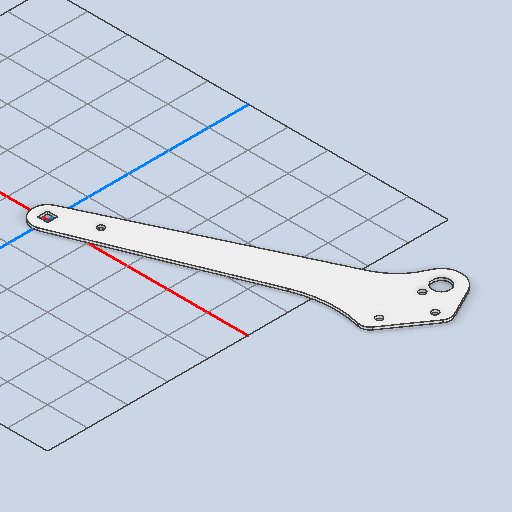
# Autodesk Inventor part: Gusset
Saved by Autodesk Inventor 2026 (Build 300175000, 175)
## iProperties
Created: 2025-04-12
Part Number: Gusset
Material: Acetal Resin, White
Document SubType Name: Modeling
Designer: avere
Density: 1.425 g/cm^3
Appearance: Smooth - White
Author: avere
Autodesk Inventor part; units mm, degrees
ref_plane "YZ Plane" through (0, 0, 0) normal (1, 0, 0) x (0, 1, 0)
ref_plane "XZ Plane" through (0, 0, 0) normal (0, 1, 0) x (-1, 0, 0)
ref_plane "XY Plane" through (0, 0, 0) normal (0, 0, 1) x (1, 0, 0)
sketch "main" plane through (0, 0, 0) normal (0, 0, 1) x (1, 0, 0)
  arc A0 (-73.5725, 33.1144) -> (-80.2841, 30.5888) centre (-75.0825, 26.9465) ccw
  circle A1 centre (-77.4831, 23.5181) radius 2.1844
  circle A2 centre (-76.8428, -4.4337) radius 2.1844
  arc A3 (-57.2294, -80.4633) -> (-56.4581, -83.5168) centre (-56.6485, -81.9407) ccw
  circle A4 centre (-92.052, 2.7116) radius 2.1844
  circle A5 centre (-78.8735, -14.4473) radius 5.5563
  line L0 (-80.2841, 30.5888) -> (-98.7239, 4.254)
  arc A6 (-98.7239, 4.254) -> (-99.1994, -2.2331) centre (-93.5223, 0.6117) ccw
  arc A7 (-90.2277, -20.1369) -> (-67.0983, -19.2049) centre (-78.8735, -14.4473) ccw
  line L1 (-99.1994, -2.2331) -> (-90.2277, -20.1369)
  arc A8 (87.2193, 64.4494) -> (80.3336, 82.1644) centre (83.1745, 73.0729) ccw
  line L2 (86.3241, 76.2225) -> (80.0249, 76.2225)
  line L3 (80.0249, 76.2225) -> (80.0249, 69.9233)
  line L4 (80.0249, 69.9233) -> (86.3241, 69.9233)
  line L5 (86.3241, 69.9233) -> (86.3241, 76.2225)
  line L6 (86.3241, 76.2225) -> (80.0249, 69.9233) construction
  line L7 (80.0249, 76.2225) -> (86.3241, 69.9233) construction
  circle A9 centre (60.3149, 62.0006) radius 2.1844
  line L8 (87.2193, 64.4494) -> (-47.8955, 1.0759)
  arc A10 (-47.8955, 1.0759) -> (-67.0983, -19.2049) centre (-31.6689, -33.5196) ccw
  line L9 (80.3336, 82.1644) -> (-32.321, 36.1639)
  arc A11 (-73.5725, 33.1144) -> (-32.321, 36.1639) centre (-57.6439, 98.1791) ccw
  point P0 (-51.4681, 8.9463)
  point P1 (-79.0426, 32.3619)
  point P2 (-100.8958, 1.1522)
  dimension "d4" = 11.1125
  dimension "d5" = 25.4
  dimension "d6" = 19.05
  dimension "d7" = 38.1
  dimension "d8" = 4.3688
  dimension "d9" = 6.35
  dimension "d10" = 25.4
  dimension "d11" = 6.35
  dimension "d12" = 6.35
  dimension "d13" = 4.3688
  dimension "d20" = 6.2992
  dimension "d21" = 6.2992
  dimension "d24" = 4.3688
  dimension "d25" = 25.4
  measures "d4" diameter of A5
  measures "d5" diameter of A7
  measures "d6" diameter of A8
  measures "d7" distance of point (-79.043, 32.362) point (-100.896, 1.152)
  measures "d8" diameter of A1
  measures "d9" distance from line of L0 A1.centre
  measures "d10" distance of A1.centre A4.centre
  measures "d11" radius of A0
  measures "d12" radius of A6
  measures "d13" diameter of A2
  measures "d20" distance of L4.end L3.end
  measures "d21" distance of L3.end L2.end
  measures "d24" diameter of A9
  measures "d25" distance of A8.centre A9.centre
sketch "Sketch1" plane through (0, 0, 0) normal (0, 1, 0) x (-1, 0, 0)
  arc A0 (-156.747, -39.9585) -> (-163.4586, -42.4842) centre (-158.257, -46.1264) ccw
  circle A1 centre (-160.6577, -49.5549) radius 2.1844
  circle A2 centre (-160.0174, -77.5067) radius 2.1844
  arc A3 (-140.4039, -153.5363) -> (-139.6326, -156.5897) centre (-139.823, -155.0137) ccw
  circle A4 centre (-175.2265, -70.3613) radius 2.1844
  circle A5 centre (-162.048, -87.5202) radius 5.5563
  line L0 (-163.4586, -42.4842) -> (-181.8985, -68.819)
  arc A6 (-181.8985, -68.819) -> (-182.3739, -75.306) centre (-176.6968, -72.4612) ccw
  arc A7 (-173.4023, -93.2099) -> (-150.2728, -92.2778) centre (-162.048, -87.5202) ccw
  line L1 (-182.3739, -75.306) -> (-173.4023, -93.2099)
  arc A8 (4.0447, -8.6236) -> (-2.8409, 9.0915) centre (0, 0) ccw
  line L2 (3.1496, 3.1496) -> (-3.1496, 3.1496)
  line L3 (-3.1496, 3.1496) -> (-3.1496, -3.1496)
  line L4 (-3.1496, -3.1496) -> (3.1496, -3.1496)
  line L5 (3.1496, -3.1496) -> (3.1496, 3.1496)
  line L6 (3.1496, 3.1496) -> (-3.1496, -3.1496) construction
  line L7 (-3.1496, 3.1496) -> (3.1496, -3.1496) construction
  circle A9 centre (-22.8596, -11.0724) radius 2.1844
  line L8 (4.0447, -8.6236) -> (-131.07, -71.997)
  arc A10 (-131.07, -71.997) -> (-150.2728, -92.2778) centre (-114.8435, -106.5926) ccw
  line L9 (-2.8409, 9.0915) -> (-115.4955, -36.9091)
  arc A11 (-156.747, -39.9585) -> (-115.4955, -36.9091) centre (-140.8184, 25.1062) ccw
  point P0 (0, 0)
extrude "Extrusion1" add sketch "Sketch1" along normal blind 1.5875
body "Solid1"
